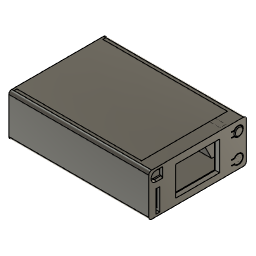
WEB-FM-Radio (Autodesk Fusion 360 design; units mm, degrees)
Autodesk Fusion 360 part; units mm, degrees
sketch "Sketch1" plane through (0, 0, 0) normal (0, 0, 1) x (1, 0, 0)
  line L0 (-38, 62.6) -> (53.5, 62.6)
  line L1 (53.5, 62.6) -> (53.5, 0)
  line L2 (53.5, 0) -> (-38, 0)
  line L3 (-38, 0) -> (-38, 62.6)
  line L4 (0, 0) -> (0, 62.6)
  line L5 (-11.5, 57.1) -> (12.5, 57.1)
  line L6 (12.5, 57.1) -> (12.5, 43.1)
  line L7 (12.5, 43.1) -> (-11.5, 43.1)
  line L8 (-11.5, 43.1) -> (-11.5, 57.1)
  circle A0 centre (33.5, 58.35) radius 2
  circle A1 centre (-33.5, 58.35) radius 2
  circle A2 centre (-33.5, 21.35) radius 2
  circle A3 centre (33.5, 21.35) radius 2
  line L9 (-33.5, 58.35) -> (33.5, 58.35) construction
  line L10 (33.5, 58.35) -> (33.5, 21.35) construction
  line L11 (33.5, 21.35) -> (-33.5, 21.35) construction
  line L12 (-33.5, 21.35) -> (-33.5, 58.35) construction
  line L13 (-40, 64.6) -> (55.5, 64.6)
  line L14 (55.5, 64.6) -> (55.5, -2)
  line L15 (55.5, -2) -> (-40, -2)
  line L16 (-40, -2) -> (-40, 64.6)
  circle A4 centre (33.5, 58.35) radius 3.5 construction
  circle A5 centre (-33.5, 58.35) radius 3.5 construction
  line L17 (-38, 0) -> (-40, 0)
  line L18 (-38, 62.6) -> (-40, 62.6)
  line L19 (41.5, 54.85) -> (30, 54.85)
  line L20 (30, 54.85) -> (30, 62.6)
  line L21 (41.5, 62.6) -> (41.5, 54.85)
  line L22 (-33.5, 39.85) -> (33.5, 39.85) construction
  line L23 (30, 17.1) -> (41.5, 17.1)
  line L24 (41.5, 17.1) -> (41.5, 24.85)
  line L25 (41.5, 24.85) -> (30, 24.85)
  line L26 (30, 24.85) -> (30, 17.1)
  line L27 (-25.5, 62.6) -> (-25.5, 54.85)
  line L28 (-38, 54.85) -> (-25.5, 54.85)
  line L29 (-25.5, 17.1) -> (-25.5, 24.85)
  line L30 (-38, 17.1) -> (-25.5, 17.1)
  line L31 (-38, 24.85) -> (-25.5, 24.85)
  dimension "d1" = 24
  dimension "d2" = 14
  dimension "d4" = 62.6
  dimension "d5" = 5.5
  dimension "d6" = 4
  dimension "d10" = 4.25
  dimension "d13" = 37
  dimension "d14" = 67
  dimension "d16" = -2
  dimension "d23" = 7
  dimension "d32" = 4.5
  dimension "d38" = 20
  dimension "d96" = 8
  dimension "d97" = 8
  dimension "d200" = 26.5
  constraint horizontal L0
  constraint vertical L1
  constraint horizontal L2
  constraint vertical L3
  constraint coincident L4.start L2
  constraint coincident L4.start origin
  constraint coincident L0 L4.end
  constraint perpendicular L0 L4
  constraint horizontal L5
  constraint vertical L6
  constraint horizontal L7
  constraint vertical L8
  constraint equal A0 A3
  constraint horizontal L9
  constraint vertical L10
  constraint horizontal L11
  constraint vertical L12
  constraint coincident A3.centre L10.end
  constraint coincident A1.centre L9.start
  constraint equal A0 A1
  constraint equal A1 A2
  constraint symmetric L4 L10 L12
  constraint coincident A0.centre L9.end
  constraint coincident A2.centre L11.end
  constraint concentric A0 A4
  constraint concentric A1 A5
  constraint equal A4 A5
  constraint coincident L16 L17.end
  constraint perpendicular L16 L17
  constraint coincident L16 L18.end
  constraint perpendicular L16 L18
  constraint horizontal L19
  constraint vertical L20
  constraint vertical L21
  constraint tangent A4 L19
  constraint tangent A4 L20
  constraint midpoint L12 L22.start
  constraint midpoint L10 L22.end
  constraint symmetric L19.start L22 L24.end
  constraint symmetric L19.end L22 L25.end
  constraint symmetric L20.end L22 L23.start
  constraint symmetric L21.start L22 L23.end
  constraint coincident L27 L28.end
  constraint perpendicular L27 L28
  constraint tangent A5 L28
  constraint symmetric L22 L28.start L31.start
  constraint symmetric L22 L27.start L29.start
  constraint symmetric L22 L27.end L29.end
  constraint coincident L0 L21.start
  constraint coincident L0 L20.end
  constraint coincident L0 L27.start
  constraint perpendicular L0 L27
  constraint coincident L3 L28.start
  constraint coincident L3 L30.start
  constraint perpendicular L3 L30
  measures "d1" distance of L6.end L7.end
  measures "d2" distance of L5.end L6.end
  measures "d4" distance of L0.start L2.end
  measures "d5" distance of L0 L5
  measures "d6" diameter of A0
  measures "d10" distance of L0 A1.centre
  measures "d13" distance of A1.centre A2.centre
  measures "d14" distance of A1.centre A0.centre
  measures "d23" diameter of A4
  measures "d32" distance of L3 A1.centre
  measures "d38" distance of L1 A0.centre
  measures "d96" distance of A0.centre L21
  measures "d97" distance of A1.centre L27
  measures "d200" distance of L3 L8
extrude "Extrude1" add sketch "Sketch1" against normal blind 1.5 contours L0 L1 L2 L13 L14 L15 L16 L17 L18 | L0 L3 L27 L28 | L3 L16 L17 L18 | L0 L2 L3 L4 L5 L7 L8 L27 L28 L29 L30 L31 | L0 L1 L2 L4 L5 L6 L7 L19 L20 L21 | L3 L29 L30 L31 | L0 L19 L20 L21 | A0 | A1 | A2 | A3 | L23 L24 L25 L26 makes body 1
extrude "Extrude2" add sketch "Sketch1" along normal blind 27.5 contours L0 L1 L2 L13 L14 L15 L16 L17 L18 bodies 1
extrude "Extrude3" add sketch "Sketch1" along normal blind 4.5 contours L0 L3 L27 L28 | L3 L29 L30 L31 | L0 L19 L20 L21 | L23 L24 L25 L26 bodies 1
chamfer "Chamfer1" distance 1 angle 45 4 edges at (12.5, 50.1, -1.5) (-11.5, 50.1, -1.5) (0.5, 57.1, -1.5) (0.5, 43.1, -1.5) on bodies 1
chamfer "Chamfer1" distance 4.5 angle 45 4 edges at (41.5, 58.725, 4.5) (41.5, 20.975, 4.5) (-25.5, 20.975, 4.5) (-25.5, 58.725, 4.5) on bodies 1
sketch "Sketch2" plane through (53.5, 0, 0) normal (-1, 0, 0) x (0, -1, 0)
  line L0 (-62.6, 0) -> (0, 0)
  line L1 (0, 0) -> (0, 27.5)
  line L2 (0, 27.5) -> (-62.6, 27.5)
  line L3 (-62.6, 27.5) -> (-62.6, 0)
  line L4 (-44.8, 4.25) -> (-17.8, 4.25)
  line L5 (-17.8, 4.25) -> (-17.8, 21.25)
  line L6 (-17.8, 21.25) -> (-44.8, 21.25)
  line L7 (-44.8, 21.25) -> (-44.8, 4.25)
  line L8 (-51.8, 12.75) -> (0, 12.75) construction
  line L9 (-56.5019, 6) -> (-54.5019, 6)
  line L10 (-59.1, 4.5) -> (-44.355, 4.5) construction
  line L11 (-56.5019, 3) -> (-54.5019, 3)
  arc A0 (-56.5019, 6) -> (-56.5019, 3) centre (-59.1, 4.5) ccw
  line L12 (-56.2804, 2.6) -> (-54.5019, 2.6)
  arc A1 (-56.2804, 6.4) -> (-56.2804, 2.6) centre (-59.1, 4.5) ccw
  line L13 (-56.2804, 6.4) -> (-54.5019, 6.4)
  line L14 (-54.5019, 6.4) -> (-54.5019, 6)
  line L15 (-54.5019, 2.6) -> (-54.5019, 3)
  line L16 (-56.2804, 22.9) -> (-54.5019, 22.9)
  arc A2 (-56.2804, 22.9) -> (-56.2804, 19.1) centre (-59.1, 21) ccw
  line L17 (-56.2804, 19.1) -> (-54.5019, 19.1)
  line L18 (-54.5019, 19.1) -> (-54.5019, 19.5)
  line L19 (-56.5019, 19.5) -> (-54.5019, 19.5)
  arc A3 (-56.5019, 22.5) -> (-56.5019, 19.5) centre (-59.1, 21) ccw
  line L20 (-56.5019, 22.5) -> (-54.5019, 22.5)
  line L21 (-54.5019, 22.9) -> (-54.5019, 22.5)
  circle A4 centre (-59.1, 4.5) radius 1.5
  circle A5 centre (-59.1, 21) radius 1.5
  arc A6 (-56.5019, 3) -> (-56.5019, 6) centre (-59.1, 4.5) ccw
  arc A7 (-56.5019, 19.5) -> (-56.5019, 22.5) centre (-59.1, 21) ccw
  line L22 (-54.5019, 19.5) -> (-54.5019, 22.5)
  line L23 (-54.5019, 3) -> (-54.5019, 6)
  line L24 (-10.8, 0) -> (-10.8, 25.5)
  line L25 (-10.8, 25.5) -> (-62.6, 25.5)
  line L26 (-52.6, 25.5) -> (-52.6, 27)
  line L27 (-52.6, 27) -> (-48.6, 27)
  line L28 (-48.6, 27) -> (-48.6, 25.5)
  line L29 (-10.8, 19.5) -> (0, 19.5)
  line L30 (-10.8, 25.5) -> (0, 25.5)
  line L31 (-2.9, 15) -> (-5.5, 15)
  line L32 (-5.5, 15) -> (-5.5, 0)
  line L33 (-10.8, 1.5) -> (-2.9, 1.5)
  line L34 (-10.8, 13.5) -> (-2.9, 13.5)
  line L35 (-7.4, 19.5) -> (-7.4, 25.5)
  line L36 (-7.4, 22.5) -> (0, 22.5) construction
  line L37 (-7.4, 20.1) -> (-2.9, 20.1)
  line L38 (-7.4, 24.9) -> (-2.9, 24.9)
  arc A8 (-2.9, 20.1) -> (-2.9, 24.9) centre (-2.9, 22.5) ccw
  line L39 (-2.9, 0) -> (-2.9, 15)
  point P0 (-59.1, 4.5)
  dimension "d33" = 27
  dimension "d34" = 17
  dimension "d48" = 4.5
  dimension "d49" = 3.5
  dimension "d50" = 6
  dimension "d51" = 3
  dimension "d52" = 2
  dimension "d53" = 0.4
  dimension "d54" = 3
  dimension "d76" = 12.75
  dimension "d125" = 25.5
  dimension "d126" = 7
  dimension "d131" = 4
  dimension "d132" = 10
  dimension "d137" = 15
  dimension "d139" = 12
  dimension "d140" = 1.5
  dimension "d143" = 51.8
  dimension "d144" = 7.4
  dimension "d146" = 4.8
  dimension "d147" = 4.5
  dimension "d149" = 6
  dimension "d150" = 2.6
  dimension "d160" = 1.5
  constraint horizontal L4
  constraint vertical L5
  constraint horizontal L6
  constraint vertical L7
  constraint symmetric L4 L6 L8
  constraint coincident P0 L10.start
  constraint horizontal L9
  constraint horizontal L10
  constraint symmetric L9.start L10 L11.start
  constraint symmetric L9.end L10 L11.end
  constraint perpendicular L9 L14
  constraint symmetric L10 L13.end L12.end
  constraint symmetric L8 L9.start L19.start
  constraint symmetric L8 L9.end L18.end
  constraint symmetric L8 L11.start A3.start
  constraint symmetric L8 L11.end L20.end
  constraint symmetric L8 A0 A3
  constraint symmetric L8 L12.start L16.start
  constraint symmetric L8 L12.end L16.end
  constraint symmetric L8 A1.start A2.end
  constraint symmetric L8 A1 A2
  constraint symmetric L8 L13.end L17.end
  constraint symmetric L8 A4 A5
  constraint symmetric L8 A6 A7
  constraint coincident L0 L24.start
  constraint perpendicular L2 L24
  constraint coincident L3 L25.end
  constraint perpendicular L3 L25
  constraint coincident L25 L26.start
  constraint perpendicular L25 L26
  constraint perpendicular L26 L27
  constraint coincident L25 L28.end
  constraint perpendicular L25 L28
  constraint coincident L24 L29.start
  constraint coincident L1 L29.end
  constraint perpendicular L1 L29
  constraint coincident L1 L30.end
  constraint perpendicular L1 L30
  constraint perpendicular L1 L31
  constraint coincident L0 L32.end
  constraint perpendicular L0 L32
  constraint perpendicular L1 L33
  constraint perpendicular L1 L34
  constraint coincident L24 L33.start
  constraint coincident L24 L34.start
  constraint coincident L29 L35.start
  constraint midpoint L35 L36.start
  constraint coincident L1 L36.end
  constraint perpendicular L1 L36
  constraint coincident L35 L37.start
  constraint perpendicular L35 L37
  constraint symmetric L36 L37.start L38.start
  constraint symmetric L36 L37.end L38.end
  constraint tangent L37 A8
  constraint coincident L30 L35.end
  constraint coincident L0 L39.start
  constraint perpendicular L8 L39
  constraint coincident L33.end L39
  constraint coincident L34.end L39
  constraint coincident L37.end L39
  measures "d33" distance of L4.start L4.end
  measures "d34" distance of L4.start L6.end
  measures "d48" distance of L0 P0
  measures "d49" distance of L3 P0
  measures "d50" diameter of A0
  measures "d51" distance of L9 L11
  measures "d52" distance of L9.start L9.end
  measures "d54" diameter of A4
  measures "d76" distance of L0 L8
  measures "d125" distance of L24.start L24.end
  measures "d126" distance of L5 L24
  measures "d131" distance of L26 L28
  measures "d132" distance of L3 L26
  measures "d137" distance of L0 L31
  measures "d139" distance of L33 L34
  measures "d140" distance of L31 L34
  measures "d143" distance of L3 L24
  measures "d144" distance of L1 L35
  measures "d146" distance of L37 L38
  measures "d147" distance of L35 A8.centre
  measures "d149" distance of L29 L30
  measures "d150" distance of L32 L39
  measures "d160" distance of L25 L27
extrude "Extrude5" cut sketch "Sketch2" against normal through all contours L0 L32 L33 L39 | L32 L33 L34 L39 | L31 L32 L34 L39 | L35 L37 L38 A8 | L4 L5 L6 L7 | L9 L11 A0 L12 A1 L13 L14 L15 | L16 A2 L17 L18 L19 A3 L20 L21 bodies 1
extrude "Extrude8" cut sketch "Sketch2" against normal up to surface (1.5 mm away) contours L9 L11 A6 L23 | L19 L20 A7 L22 bodies 1
extrude "Extrude22" add sketch "Sketch2" along normal blind 7 contours L0 L24 L32 L33 | L1 L2 L3 L25 L26 L27 L28 L30 | L0 L32 L33 L39 | L0 L1 L24 L29 L31 L32 L34 L39 | L31 L32 L34 L39 bodies 1
extrude "Extrude34" cut 2 faces at (53.5, 4.6333, 1) (53.5, 3.7667, 14.5) along direction (-1, 0, 0) blind 5 on bodies 1 bodies 1
chamfer "Chamfer3" distance 1.5 angle 45 4 edges at (55.5, 44.8, 12.75) (55.5, 31.3, 21.25) (55.5, 17.8, 12.75) (55.5, 31.3, 4.25) on bodies 1
chamfer "Chamfer3" distance 1 angle 45 3 edges at (55.5, 5.15, 20.1) (55.5, 0.5, 22.5) (55.5, 5.15, 24.9) on bodies 1
sketch "Sketch3" plane through (0, 64.6, 0) normal (0, -1, 0) x (1, 0, 0)
  line L0 (52, 17.25) -> (53.5, 17.25)
  line L1 (54.5, 16.25) -> (54.5, 9.25)
  line L2 (53.5, 8.25) -> (52, 8.25)
  line L3 (51, 9.25) -> (51, 16.25)
  line L4 (55.5, 27.5) -> (55.5, -1.5)
  line L5 (55.5, -1.5) -> (-40, -1.5)
  line L6 (-40, -1.5) -> (-40, 27.5)
  line L7 (-40, 27.5) -> (55.5, 27.5)
  arc A0 (54.5, 16.25) -> (53.5, 17.25) centre (53.5, 16.25) ccw
  arc A1 (52, 17.25) -> (51, 16.25) centre (52, 16.25) ccw
  arc A2 (51, 9.25) -> (52, 8.25) centre (52, 9.25) ccw
  arc A3 (53.5, 8.25) -> (54.5, 9.25) centre (53.5, 9.25) ccw
  circle A4 centre (49, 24.5) radius 0.75
  line L8 (53.5, 25.5) -> (46.5, 25.5)
  point P0 (51, 17.25)
  point P1 (54.5, 17.25)
  point P2 (51, 8.25)
  point P3 (53.5, 0)
  dimension "d39" = 3.5
  dimension "d40" = 9
  dimension "d44" = 8.25
  dimension "d45" = 1
  dimension "d123" = 1
  dimension "d257" = 1.5
  dimension "d258" = 2
  dimension "d259" = 1
  constraint horizontal L0
  constraint vertical L1
  constraint horizontal L2
  constraint vertical L3
  constraint coincident P1 L0
  constraint coincident P1 L1
  constraint tangent L0 A0
  constraint tangent L1 A0
  constraint coincident P0 L0
  constraint coincident P0 L3
  constraint tangent L0 A1
  constraint tangent L3 A1
  constraint equal A0 A1
  constraint coincident P2 L2
  constraint coincident P2 L3
  constraint tangent L2 A2
  constraint tangent L3 A2
  constraint equal A0 A2
  constraint tangent L1 A3
  constraint tangent L2 A3
  constraint equal A0 A3
  measures "d39" distance of P0 P1
  measures "d40" distance of P0 P2
  measures "d44" distance of L2 P3
  measures "d45" radius of A0
  measures "d123" distance of L1 L4
  measures "d257" diameter of A4
  measures "d258" distance of L3 A4.centre
  measures "d259" distance of A4.centre L8
extrude "Extrude6" cut sketch "Sketch3" along normal blind 8 contours L0 L1 L2 L3 A0 A1 A2 A3 | A4 bodies 1
extrude "Extrude10" cut sketch "Sketch2" along normal blind -1.5 and the other way blind 1 contours A4 | A5 bodies 1
ref_plane "WorkPlane1" through (-38.5, 31.3, 13) normal (-1, 0, 0) x (0, 1, 0)
sketch "Sketch4" plane through (-38.5, 31.3, 13) normal (-1, 0, 0) x (0, -1, 0)
  line L0 (31.3, -13) -> (31.3, 14.5)
  line L1 (-31.3, -13) -> (-31.3, 14.5)
  line L2 (-33.3, -14.5) -> (-33.3, 14.5)
  line L3 (33.3, 14.5) -> (33.3, -14.5)
  line L4 (33.3, -14.5) -> (-33.3, -14.5)
  line L5 (33.3, 14.5) -> (-33.3, 14.5)
  line L6 (-31.3, 12.5) -> (31.3, 12.5)
  line L7 (-31.3, -13) -> (31.3, -13)
  line L8 (31.3, 13.5) -> (-31.3, 13.5)
  line L9 (-31.3, -8.5) -> (-23.55, -8.5)
  circle A0 centre (-14.4827, 6.3) radius 2.7
  line L10 (-1.6827, 12.5) -> (-1.6827, 6.3)
  line L11 (-1.6827, 10.5) -> (-27.2827, 10.5)
  line L12 (-27.2827, 6.3) -> (-27.2827, 12.5)
  line L13 (-6.4827, 10.5) -> (-6.4827, 12.5)
  line L14 (-22.4827, 10.5) -> (-22.4827, 12.5)
  line L15 (-27.2827, 6.3) -> (-31.3, 6.3)
  line L16 (-1.6827, 6.3) -> (31.3, 6.3)
  line L17 (-1.6827, 8.7) -> (-2.6827, 8.7)
  line L18 (-2.6827, 8.7) -> (-2.6827, 6.3)
  line L19 (-2.6827, 6.3) -> (-1.6827, 6.3)
  line L20 (-27.2827, 8.7) -> (-26.2827, 8.7)
  line L21 (-26.2827, 8.7) -> (-26.2827, 6.3)
  line L22 (-26.2827, 6.3) -> (-27.2827, 6.3)
  line L23 (-29.3, 13.5) -> (-29.3, 14.5)
  line L24 (29.3, 13.5) -> (29.3, 14.5)
  circle A1 centre (5.3173, 8.8) radius 3.1
  line L25 (11.3173, 6.3) -> (11.3173, 11.3)
  line L26 (11.3173, 11.3) -> (-0.6827, 11.3)
  line L27 (-0.6827, 11.3) -> (-0.6827, 6.3)
  line L28 (11.3173, 8.8) -> (-0.6827, 8.8) construction
  line L29 (5.3173, 11.3) -> (5.3173, 6.3) construction
  line L30 (-14.4827, 6.3) -> (-14.4827, 10.5) construction
  line L31 (-27.2913, 6.3) -> (-27.2913, 3.3)
  line L32 (-26.2827, 3.3) -> (-31.3, 3.3)
  line L33 (-28.7913, 3.3) -> (-28.7913, 6.3) construction
  line L34 (-27.5413, 3.3) -> (-27.5413, 6.8)
  line L35 (-30.0413, 3.3) -> (-30.0413, 6.8)
  line L36 (-27.5413, 6.8) -> (-30.0413, 6.8)
  line L37 (-30.2913, 3.3) -> (-30.2913, 6.3)
  line L38 (-29.5413, 3.3) -> (-29.5413, 6.3)
  line L39 (-28.0413, 3.3) -> (-28.0413, 6.3)
  line L40 (12.3173, 6.3) -> (12.3173, 12.5)
  line L41 (30.3, 6.3) -> (30.3, 12.5)
  line L42 (-26.2827, 6.3) -> (-26.2827, 3.3)
  line L43 (0.8173, 6.3) -> (0.8173, 11.3)
  line L44 (9.8173, 6.3) -> (9.8173, 11.3)
  circle A2 centre (21.8, 3.25) radius 9.25
  point P0 (-27.05, -13)
  dimension "d77" = 2
  dimension "d151" = 4.2
  dimension "d152" = 25.6
  dimension "d153" = 16
  dimension "d154" = 2
  dimension "d157" = 1
  dimension "d158" = 1.8
  dimension "d172" = 2
  dimension "d178" = 2
  dimension "d179" = 1
  dimension "d206" = 6.2
  dimension "d207" = 12
  dimension "d208" = 5
  dimension "d209" = 1
  dimension "d223" = 2.5
  dimension "d224" = 0.5
  dimension "d225" = 3
  dimension "d226" = 3
  dimension "d232" = 1.5
  dimension "d234" = 5.4
  dimension "d238" = 1
  dimension "d248" = 9
  dimension "d251" = 18.5
  dimension "d254" = 11.5
  constraint coincident L3.start L5.start
  constraint coincident L2.end L5.end
  constraint coincident L1 L6.start
  constraint coincident L0 L6.end
  constraint perpendicular L0 L6
  constraint coincident L1.start L7.start
  constraint coincident L0.start L7.end
  constraint coincident L1 L8.end
  constraint perpendicular L1 L8
  constraint coincident L6 L10.start
  constraint perpendicular L6 L10
  constraint perpendicular L10 L11
  constraint coincident L6 L12.end
  constraint perpendicular L6 L12
  constraint coincident L11 L13.start
  constraint coincident L6 L13.end
  constraint perpendicular L6 L13
  constraint coincident L12 L11.end
  constraint coincident L1 L15.end
  constraint perpendicular L1 L15
  constraint coincident A0.centre L15
  constraint coincident L11.start L10
  constraint coincident L15 L10.end
  constraint coincident L0 L16.end
  constraint perpendicular L0 L16
  constraint coincident L10 L17.start
  constraint perpendicular L10 L17
  constraint perpendicular L17 L18
  constraint coincident L10 L16.start
  constraint perpendicular L10 L19
  constraint coincident L10.end L16.start
  constraint coincident L5 L23.end
  constraint perpendicular L5 L23
  constraint coincident L5 L24.end
  constraint perpendicular L5 L24
  constraint coincident L0 L8.start
  constraint coincident L23.start L8
  constraint coincident L8 L24.start
  constraint coincident L16 L25.start
  constraint perpendicular L16 L25
  constraint perpendicular L25 L26
  constraint coincident L16 L27.end
  constraint perpendicular L16 L27
  constraint midpoint L25 L28.start
  constraint midpoint L27 L28.end
  constraint midpoint L26 L29.start
  constraint coincident L16 L29.end
  constraint perpendicular L16 L29
  constraint midpoint A1.centre L29
  constraint coincident L12 L20.start
  constraint coincident L12 L15.start
  constraint coincident A0.centre L30.start
  constraint midpoint L11 L30.end
  constraint symmetric L18 L21 L30
  constraint symmetric L19 L22 L30
  constraint symmetric L17 L20 L30
  constraint perpendicular L12 L22
  constraint symmetric L13 L14 L30
  constraint coincident L6 L14.end
  constraint coincident L11 L14.start
  constraint coincident L15 L31.start
  constraint perpendicular L15 L31
  constraint perpendicular L1 L32
  constraint midpoint L32 L33.start
  constraint coincident L15 L33.end
  constraint perpendicular L15 L33
  constraint coincident L32 L34.start
  constraint perpendicular L15 L34
  constraint coincident L32 L35.start
  constraint perpendicular L15 L35
  constraint perpendicular L34 L36
  constraint coincident L15 L37.end
  constraint perpendicular L15 L37
  constraint coincident L32 L31.end
  constraint coincident L1 L32.end
  constraint coincident L32 L38.start
  constraint coincident L15 L38.end
  constraint perpendicular L15 L38
  constraint symmetric L33 L38.start L39.start
  constraint symmetric L33 L38.end L39.end
  constraint coincident L16 L41.start
  constraint coincident L16 L40.start
  constraint coincident L6 L40.end
  constraint perpendicular L6 L40
  constraint coincident L6 L41.end
  constraint perpendicular L6 L41
  constraint perpendicular L32 L42
  constraint coincident L16 L43.start
  constraint coincident L26 L43.end
  constraint perpendicular L26 L43
  constraint symmetric L29 L43.start L44.start
  constraint symmetric L29 L43.end L44.end
  constraint tangent L6 A2
  measures "d77" distance of L5 L6
  measures "d151" distance of A0.centre L11
  measures "d152" distance of L10 L12
  measures "d153" distance of L13 L14
  measures "d154" distance of L6 L11
  measures "d157" distance of L10 L18
  measures "d158" distance of L11 L17
  measures "d172" distance of L23.start L8.end
  measures "d178" distance of L0 L24.start
  measures "d179" distance of L5 L8
  measures "d206" diameter of A1
  measures "d207" distance of L25.end L26.end
  measures "d208" distance of L25.start L25.end
  measures "d209" distance of L10 L27
  measures "d223" distance of L34 L35
  measures "d224" distance of L15 L36
  measures "d225" distance of L31 L37
  measures "d226" distance of L31.start L31.end
  measures "d232" distance of L38 L39
  measures "d234" diameter of A0
  measures "d238" distance of L25 L40
  measures "d248" distance of L43 L44
  measures "d251" diameter of A2
  measures "d254" distance of L3 A2.centre
extrude "Extrude12" add sketch "Sketch4" along normal up to surface (1.5 mm away) separate body contours L0 L1 L7 L10 L11 L12 L16 L17 L18 L19 L20 L21 A1 L32 L42 A2 | L0 L6 L16 L41 A2 | L0 L1 L6 L8 | L16 A2 | L16 L41 A2 | L0 L5 L8 L24 | L6 L41 A2 | L16 L41 A2 | L1 L15 L32 L37 | L5 L8 L23 L24 | L6 L16 L40 A2 | L1 L6 L12 L15 L34 L35 L36 | L1 L5 L8 L23 | L6 L10 L16 A1 L25 L26 L27 L40 | L6 L10 L11 L13 | L16 L25 L26 L44 | L6 L11 L12 L14 | L15 L34 L35 L36 | L6 L11 L13 L14 | L16 A1 L26 L44 | L10 L17 L18 L19 | L12 L20 L21 L22 | L16 A1 L26 L43 | L15 L22 L31 L32 L42 | L16 L26 L27 L43 | A0 makes body 2
extrude "Extrude28" add sketch "Sketch4" against normal up to surface (85 mm away) contours L5 L8 L23 L24 bodies 2
extrude "Extrude29" add sketch "Sketch4" against normal up to surface (83 mm away) contours L0 L1 L6 L8 bodies 2
extrude "Extrude24" add sketch "Sketch4" against normal blind 40 contours L0 L6 L16 L41 A2 | L6 L41 A2 | L6 L16 L40 A2 | L1 L6 L12 L15 L34 L35 L36 | L6 L10 L16 A1 L25 L26 L27 L40 | L16 L25 L26 L44 | L15 L34 L35 L36 | L6 L11 L13 L14 | L10 L17 L18 L19 | L12 L20 L21 L22 | L16 L26 L27 L43 bodies 2
extrude "Extrude40" cut sketch "Sketch4" against normal blind 15 contours L16 L25 L26 L44 | L16 L26 L27 L43 bodies 2
extrude "Extrude35" add sketch "Sketch4" against normal blind 10 contours L1 L15 L32 L37 | L15 L32 L35 L37 | L15 L32 L35 L38 | L15 L34 L35 L36 | L15 L32 L38 L39 | L15 L32 L34 L39 | L15 L31 L32 L34 | L15 L22 L31 L32 L42 bodies 2
extrude "Extrude25" add sketch "Sketch4" against normal up to surface (85 mm away) contours L0 L5 L8 L24 | L1 L5 L8 L23 bodies 1
sketch "Sketch5" plane through (46.5, 0, 0) normal (-1, 0, 0) x (0, -1, 0)
  line L0 (-52.6, 25.5) -> (-52.6, 27)
  line L1 (-52.6, 27) -> (-48.6, 27)
  line L2 (-48.6, 27) -> (-48.6, 25.5)
  line L3 (-48.6, 25.5) -> (0, 25.5)
  line L4 (0, 25.5) -> (0, 26.5)
  line L5 (-2, 27.5) -> (-60.6, 27.5)
  line L6 (-62.6, 26.5) -> (-62.6, 25.5)
  line L7 (-62.6, 26.5) -> (-52.6, 26.5)
  line L8 (-60.6, 26.5) -> (0, 26.5)
  line L9 (-62.6, 25.5) -> (-52.6, 25.5)
  line L10 (-2, 26.5) -> (-2, 27.5)
  line L11 (-60.6, 27.5) -> (-60.6, 26.5)
  line L12 (-60.6, 26.5) -> (-62.6, 26.5)
  line L13 (0, 26.5) -> (-2, 26.5)
  line L14 (-62.6, 25.5) -> (0, 25.5)
  constraint coincident L0 L7.end
  constraint perpendicular L0 L7
  constraint coincident L4.end L8.end
  constraint perpendicular L4 L8
  constraint coincident L8.start L11.end
extrude "Extrude30" add sketch "Sketch5" along normal blind 2 contours L0 L6 L7 L8 L9 L12 L14 | L2 L3 L4 L8 L13 L14 bodies 1
sketch "Sketch6" plane through (-40, 0, 0) normal (-1, 0, 0) x (0, -1, 0)
  line L0 (-62.6, 27.5) -> (-62.6, 0)
  line L1 (-62.6, 0) -> (0, 0)
  line L2 (0, 0) -> (0, 27.5)
  line L3 (0, 27.5) -> (-62.6, 27.5)
  circle A0 centre (-25.9827, 21.8) radius 3.1
  line L4 (-61.5913, 19.3) -> (-58.5913, 19.3)
  line L5 (-58.5913, 16.3) -> (-61.5913, 16.3)
  line L6 (-61.5913, 16.3) -> (-61.5913, 19.3)
  line L7 (-58.5913, 19.3) -> (-58.5913, 16.3)
extrude "Extrude31" add sketch "Sketch2" against normal blind 1 separate body contours A3 A7 | A5 makes body 3
extrude "Extrude32" add sketch "Sketch2" along normal blind 0.5 contours A5 bodies 3
chamfer "Chamfer8" distance 0.5 angle 45 1 edges at (54.5, 60.9798, 23.338) on bodies 3
move_body "Move1" bodies 3 to x (1, 0, 0) y (0, 1, 0) z (0, 0, 1) at (1.5, 0, 0)
sketch "Sketch7" plane through (1.5, 0, 0) normal (1, 0, 0) x (0, 1, 0)
  line L0 (58.5827, 25.5) -> (58.5827, 21.7)
  line L1 (58.5827, 21.7) -> (57.5827, 21.7)
  line L2 (57.5827, 21.7) -> (57.5827, 19.3)
  line L3 (57.5827, 19.3) -> (62.6, 19.3)
  line L4 (62.6, 19.3) -> (62.6, 25.5)
  line L5 (62.6, 25.5) -> (58.5827, 25.5)
  line L6 (62.6, 23.5) -> (60.6, 23.5)
  line L7 (60.6, 23.5) -> (60.6, 25.5)
  line L8 (0, 23.5) -> (2, 23.5)
  line L9 (2, 23.5) -> (2, 25.5)
  line L10 (0, 25.5) -> (62.6, 25.5)
  line L11 (0, 25.5) -> (0, 19.3)
  dimension "d194" = 2
  dimension "d195" = 2
  constraint coincident L4 L6.start
  constraint perpendicular L4 L6
  constraint coincident L5 L7.end
  constraint perpendicular L5 L7
  constraint horizontal L8
  constraint perpendicular L8 L9
  constraint coincident L9.end L10
  constraint coincident L8.start L11
  constraint equal L6 L8
  constraint equal L7 L9
  measures "d194" distance of L6.start L6.end
  measures "d195" distance of L6.end L7.end
extrude "Extrude33" add sketch "Sketch7" along normal blind 15 contours L4 L5 L6 L7 L10 | L8 L9 L10 L11 bodies 1
chamfer "Chamfer9" distance 2 angle 45 2 edges at (16.5, 60.6, 24.5) (16.5, 2, 24.5) on bodies 1
chamfer "Chamfer9" distance 1 angle 45 2 edges at (1.5, 1, 25.5) (1.5, 61.6, 25.5) on bodies 1
fillet "Fillet1" radius 2 4 edges at (7.75, -2, 27.5) (7.75, -2, -1.5) (7.75, 64.6, -1.5) (7.75, 64.6, 27.5) on bodies 1
extrude "Extrude36" cut sketch "Sketch4" against normal blind 8.5 contours L15 L32 L35 L38 | L15 L34 L35 L36 | L15 L32 L38 L39 | L15 L32 L34 L39 bodies 2
extrude "Extrude37" cut sketch "Sketch4" against normal through all contours L15 L32 L38 L39 bodies 2
chamfer "Chamfer14" distance 4 angle 45 4 edges at (1.5, 60.0913, 19.3) (1.5, 0.3837, 19.3) (1.5, 19.8577, 19.3) (1.5, 32.2327, 19.3) on bodies 2
chamfer "Chamfer14" distance 10 angle 45 3 edges at (-38.5, 0.3837, 19.3) (-38.5, 19.1077, 19.3) (-38.5, 32.9827, 19.3) on bodies 2
equation "d44 = ( 25.5 mm - d40 ) / 2"
equation "d97 = d96"
named bodies: "case", "cover", "button"
